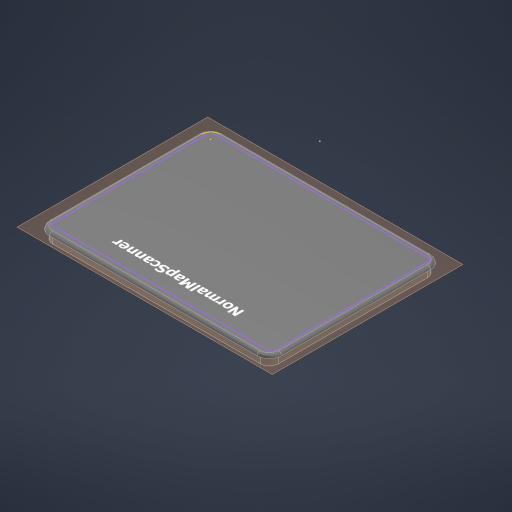
# Autodesk Inventor part: board_box_cover
Saved by Autodesk Inventor 2023 (Build 270158030, 158C)
## iProperties
Created: 2022-07-16
Part Number: board_box_cover
Material: Thermoplastic Resin
Document SubType Name: Modeling
Designer: Norbert Ligas
Density: 1.28 g/cm^3
Appearance: Smooth - Black
Mass: 94.9977 g
Surface Area: 403.961 cm^2
Volume: 74.2169 cm^3
Author: Norbert Ligas
Autodesk Inventor part; units mm, degrees
ref_plane "YZ Plane" through (0, 0, 0) normal (1, 0, 0) x (0, 1, 0)
ref_plane "XZ Plane" through (0, 0, 0) normal (0, 1, 0) x (-1, 0, 0)
ref_plane "XY Plane" through (0, 0, 0) normal (0, 0, 1) x (1, 0, 0)
ref_plane "Work Plane1" through (30.9658, 19.9385, 83.0324) normal (0, 1, 0) x (-1, 0, 0)
sketch "Sketch1" plane through (30.9658, 19.9385, 83.0324) normal (0, 1, 0) x (-1, 0, 0)
  line L0 (-67.65, -52.5) -> (67.65, -52.5) projected
  arc A0 (67.65, -52.5) -> (71.65, -48.5) centre (67.65, -48.5) ccw projected
  line L1 (71.65, -48.5) -> (71.65, 48.5) projected
  arc A1 (71.65, 48.5) -> (67.65, 52.5) centre (67.65, 48.5) ccw projected
  line L2 (67.65, 52.5) -> (-67.65, 52.5) projected
  arc A2 (-67.65, 52.5) -> (-71.65, 48.5) centre (-67.65, 48.5) ccw projected
  line L3 (-71.65, 48.5) -> (-71.65, -48.5) projected
  arc A3 (-71.65, -48.5) -> (-67.65, -52.5) centre (-67.65, -48.5) ccw projected
  arc A4 (-73.65, -48.5) -> (-67.65, -54.5) centre (-67.65, -48.5) ccw projected
  line L4 (-73.65, -48.5) -> (-73.65, 48.5) projected
  arc A5 (-67.65, 54.5) -> (-73.65, 48.5) centre (-67.65, 48.5) ccw projected
  line L5 (-67.65, 54.5) -> (67.65, 54.5) projected
  arc A6 (73.65, 48.5) -> (67.65, 54.5) centre (67.65, 48.5) ccw projected
  line L6 (73.65, 48.5) -> (73.65, -48.5) projected
  arc A7 (67.65, -54.5) -> (73.65, -48.5) centre (67.65, -48.5) ccw projected
  line L7 (67.65, -54.5) -> (-67.65, -54.5) projected
  arc A8 (-75.65, -48.5) -> (-67.65, -56.5) centre (-67.65, -48.5) ccw projected
  line L8 (-75.65, 48.5) -> (-75.65, -48.5) projected
  arc A9 (-67.65, 56.5) -> (-75.65, 48.5) centre (-67.65, 48.5) ccw projected
  line L9 (67.65, 56.5) -> (-67.65, 56.5) projected
  arc A10 (75.65, 48.5) -> (67.65, 56.5) centre (67.65, 48.5) ccw projected
  line L10 (75.65, -48.5) -> (75.65, 48.5) projected
  arc A11 (67.65, -56.5) -> (75.65, -48.5) centre (67.65, -48.5) ccw projected
  line L11 (-67.65, -56.5) -> (67.65, -56.5) projected
  point P0 (30.9658, -83.0324)
extrude "Extrusion1" add sketch "Sketch1" along normal blind 2 contours A3 L3 A2 L2 A1 L1 A0 L0 | L4 A5 L5 A6 L6 A7 L7 A4 | L8 A9 L9 A10 L10 A11 L11 A8
sketch "Sketch2" plane through (30.9658, 19.9385, 83.0324) normal (0, -1, 0) x (1, 0, 0)
  arc A0 (-67.65, 54.5) -> (-73.65, 48.5) centre (-67.65, 48.5) ccw projected
  arc A1 (-67.65, 54.5) -> (-73.65, 48.5) centre (-67.65, 48.5) ccw projected
  line L0 (67.65, 54.5) -> (-67.65, 54.5) projected
  line L1 (-67.65, 54.5) -> (67.65, 54.5) projected
  arc A2 (73.65, 48.5) -> (67.65, 54.5) centre (67.65, 48.5) ccw projected
  arc A3 (73.65, 48.5) -> (67.65, 54.5) centre (67.65, 48.5) ccw projected
  line L2 (73.65, -48.5) -> (73.65, 48.5) projected
  line L3 (73.65, 48.5) -> (73.65, -48.5) projected
  arc A4 (67.65, -54.5) -> (73.65, -48.5) centre (67.65, -48.5) ccw projected
  arc A5 (67.65, -54.5) -> (73.65, -48.5) centre (67.65, -48.5) ccw projected
  line L4 (67.65, -54.5) -> (-67.65, -54.5) projected
  line L5 (-67.65, -54.5) -> (67.65, -54.5) projected
  line L6 (-73.65, 48.5) -> (-73.65, -48.5) projected
  line L7 (-73.65, -48.5) -> (-73.65, 48.5) projected
  arc A6 (-73.65, -48.5) -> (-67.65, -54.5) centre (-67.65, -48.5) ccw projected
  arc A7 (-73.65, -48.5) -> (-67.65, -54.5) centre (-67.65, -48.5) ccw projected
  line L8 (-67.65, 52.5) -> (67.65, 52.5) projected
  arc A8 (-67.65, 52.5) -> (-71.5036, 49.5724) centre (-67.65, 48.5) ccw projected
  line L9 (-71.65, -38) -> (-71.65, 38) projected
  line L10 (71.65, 48.5) -> (71.65, -48.5) projected
  arc A9 (71.65, 48.5) -> (67.65, 52.5) centre (67.65, 48.5) ccw projected
  line L11 (-67.65, 52.5) -> (67.65, 52.5) projected
  line L12 (71.65, 48.5) -> (71.65, -48.5) projected
  arc A10 (67.65, -52.5) -> (71.65, -48.5) centre (67.65, -48.5) ccw projected
  line L13 (67.65, -52.5) -> (-67.65, -52.5) projected
  arc A11 (-71.65, -48.5) -> (-67.65, -52.5) centre (-67.65, -48.5) ccw projected
  line L14 (-71.65, -43) -> (-71.65, -47.5) projected
  line L15 (-71.65, -40.4) -> (-71.65, -38) projected
  line L16 (-71.65, -38) -> (-71.65, 38) projected
  line L17 (-71.65, -38) -> (-71.65, 38) projected
  circle A12 centre (-67.65, 48.5) radius 4
  circle A13 centre (-67.65, -48.5) radius 4
  circle A14 centre (67.65, -48.5) radius 4
  circle A15 centre (67.65, 48.5) radius 4
  line L18 (67.65, 52.5) -> (-67.65, 52.5)
  line L19 (-71.65, 48.5) -> (-71.65, -48.5)
  line L20 (-67.65, -52.5) -> (67.65, -52.5)
  line L21 (71.65, -48.5) -> (71.65, 48.5)
  point P0 (-30.9658, -83.0324)
  point P1 (-67.65, 54.5)
  point P2 (-73.65, 48.5)
  point P3 (-71.5036, 49.5724)
  constraints: 8 end point, 4 coincident, 4 tangent, 3 centre point, 2 collinear, 2 concentric, 2 point on circle, 1 horizontal, 1 perpendicular, 1 vertical, 1 vertical alignment, 2 other
extrude "Extrusion2" add sketch "Sketch2" along normal blind 6
sketch "Sketch4" plane through (30.9658, 19.9385, 83.0324) normal (0, -1, 0) x (1, 0, 0)
  arc A0 (-67.65, 54.5) -> (-73.65, 48.5) centre (-67.65, 48.5) ccw projected
  arc A1 (-73.65, -48.5) -> (-67.65, -54.5) centre (-67.65, -48.5) ccw projected
  line L0 (67.65, -54.5) -> (-67.65, -54.5) projected
  arc A2 (67.65, -54.5) -> (73.65, -48.5) centre (67.65, -48.5) ccw projected
  line L1 (-73.65, -48.5) -> (-73.65, 48.5) projected
  line L2 (-67.65, 54.5) -> (67.65, 54.5) projected
  arc A3 (73.65, 48.5) -> (67.65, 54.5) centre (67.65, 48.5) ccw projected
  line L3 (73.65, 48.5) -> (73.65, -48.5) projected
  point P0 (-30.9658, -83.0324)
extrude "Extrusion3" add sketch "Sketch4" along normal blind 2
sketch "Sketch6" plane through (30.9658, 17.9385, 83.0324) normal (0, -1, 0) x (1, 0, 0)
  circle A0 centre (30.75, -29) radius 1.375 projected
  circle A1 centre (-18.25, -29) radius 1.375 projected
  circle A2 centre (30.75, 29) radius 1.375 projected
  circle A3 centre (-18.25, 29) radius 1.375 projected
  circle A4 centre (30.75, -29) radius 1.25
  circle A5 centre (30.75, 29) radius 1.25
  circle A6 centre (-18.25, 29) radius 1.25
  circle A7 centre (-18.25, -29) radius 1.25
  circle A8 centre (30.75, -29) radius 3.25
  circle A9 centre (-18.25, -29) radius 3.25
  circle A10 centre (-18.25, 29) radius 3.25
  circle A11 centre (30.75, 29) radius 3.25
  point P0 (-30.9658, -83.0324)
  dimension "d6" = 2.5
  dimension "d7" = 2
  constraints: 8 centre point, 8 coincident, 6 equal radius
  measures "d6" diameter of A4
  measures "d7" radial gap between concentric circles of A4 A8
extrude "Extrusion4" add sketch "Sketch6" along normal blind 15 contours A0 | A1 | A2 | A3 | A4 | A5 | A6 | A7 | A8 | A9 | A10 | A11
sketch "Sketch7" plane through (61.7158, 2.9385, 54.0324) normal (0, -1, 0) x (1, 0, 0)
  circle A0 centre (0, 0) radius 3.25 projected
  circle A1 centre (-49, 58) radius 3.25 projected
  circle A2 centre (-49, 0) radius 3.25 projected
  circle A3 centre (0, 58) radius 3.25 projected
  circle A4 centre (0, 0) radius 3.25 projected
  circle A5 centre (0, 0) radius 1.25
  circle A6 centre (-49, 0) radius 1.25
  circle A7 centre (-49, 58) radius 3.25 projected
  circle A8 centre (-49, 58) radius 1.25
  circle A9 centre (0, 58) radius 1.25
  dimension "d10" = 2
  dimension "d11" = 2.5
  constraints: 4 centre point, 4 coincident, 3 equal radius
  measures "d10" radial gap between concentric circles of A0 A5
  measures "d11" diameter of A5
extrude "Extrusion5" add sketch "Sketch7" along normal blind 7
fillet "Fillet1" radius 2 8 edges at (30.9658, 21.9385, 139.5324) (104.2726, 21.9385, 137.1892) (106.6158, 21.9385, 83.0324) (104.2726, 21.9385, 28.8755) (30.9658, 21.9385, 26.5324) (-42.3411, 21.9385, 28.8755) (-44.6842, 21.9385, 83.0324) (-42.3411, 21.9385, 137.1892)
fillet "Fillet2" radius 0.5 16 edges at (-42.6842, 13.9385, 83.0324) (-40.9269, 13.9385, 30.2897) (30.9658, 13.9385, 28.5324) (102.8584, 13.9385, 30.2897) (104.6158, 13.9385, 83.0324) (102.8584, 13.9385, 135.775) (30.9658, 13.9385, 137.5324) (-40.9269, 13.9385, 135.775) (-39.5127, 13.9385, 134.3608) (30.9658, 13.9385, 135.5324) (101.4442, 13.9385, 134.3608) (102.6158, 13.9385, 83.0324) (101.4442, 13.9385, 31.7039) (30.9658, 13.9385, 30.5324) (-39.5127, 13.9385, 31.7039) (-40.6842, 13.9385, 83.0324)
fillet "Fillet3" radius 0.5 8 edges at (58.4658, -4.0615, 54.0324) (60.4658, -4.0615, 54.0324) (9.4658, -4.0615, 54.0324) (11.4658, -4.0615, 54.0324) (9.4658, -4.0615, 112.0324) (11.4658, -4.0615, 112.0324) (58.4658, -4.0615, 112.0324) (60.4658, -4.0615, 112.0324)
fillet "Fillet4" radius 4 12 edges at (101.4442, 17.9385, 31.7039) (30.9658, 17.9385, 30.5324) (-39.5127, 17.9385, 31.7039) (-40.6842, 17.9385, 83.0324) (-39.5127, 17.9385, 134.3608) (30.9658, 17.9385, 135.5324) (101.4442, 17.9385, 134.3608) (102.6158, 17.9385, 83.0324) (58.4658, 17.9385, 112.0324) (9.4658, 17.9385, 112.0324) (58.4658, 17.9385, 54.0324) (9.4658, 17.9385, 54.0324)
sketch "Sketch8" plane through (30.9658, 21.9385, 83.0324) normal (0, 1, 0) x (1, 0, 0)
  line L0 (20.0468, -46.746) -> (-21.1449, -46.746) construction
  line L1 (-21.1449, -46.746) -> (-21.1449, -32.5377) construction
  line L2 (-21.1449, -32.5377) -> (20.0468, -32.5377) construction
  line L3 (20.0468, -32.5377) -> (20.0468, -46.746) construction
  arc A0 (-67.65, 54.5) -> (-73.65, 48.5) centre (-67.65, 48.5) ccw projected
  line L4 (72.15, -51.7421) -> (-71.9714, -51.7421)
  line L5 (-71.9714, -51.7421) -> (-71.9714, 52.6624)
  line L6 (-71.9714, 52.6624) -> (72.15, 52.6624)
  line L7 (72.15, 52.6624) -> (72.15, -51.7421)
  point P0 (-30.9658, 83.0324)
  constraints: 8 end point, 2 parallel, 1 horizontal, 1 perpendicular, 1 point on circle, 2 other
equation "\"d0\" = 0.5 * cover_thickness"
equation "\"d2\" = 1.5 * cover_thickness"
equation "\"d4\" = 0.5 * cover_thickness"
equation "\"d6\" = spacer_thread_diameter"
equation "\"d7\" = stabilizer_wall_thickness"
equation "\"d8\" = measure_spacer_to_cover_distance"
equation "\"d10\" = stabilizer_wall_thickness"
equation "\"d12\" = spacer_thread_length"
equation "\"cover_thickness\" = 4"
equation "\"spacer_thread_diameter\" = 2.5"
equation "\"stabilizer_length_tolerance_subtraction\" = 1"
equation "\"spacer_thread_length_tolerance_addition\" = 2"
equation "\"stabilizer_wall_thickness\" = 2"
equation "\"text_grave_depth\" = 1"
equation "\"measure_spacer_to_cover_distance\" = 15"
equation "\"spacer_thread_length\" = 7"
body "Solid1"
